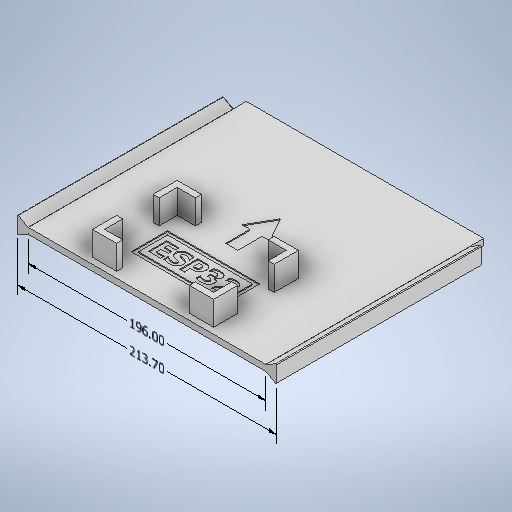
# Autodesk Inventor part: Suelo2
Saved by Autodesk Inventor 2025.1 (Build 291241000, 241)
## iProperties
Created: 2025-11-20
Part Number: Suelo2
Material: Genérico
Document SubType Name: Modeling
Designer: Diego
Density: 1 g/cm^3
Appearance: Valor por defecto
Author: Diego
Autodesk Inventor part; units mm, degrees
ref_plane "YZ Plane" through (0, 0, 0) normal (1, 0, 0) x (0, 1, 0)
ref_plane "XZ Plane" through (0, 0, 0) normal (0, 1, 0) x (-1, 0, 0)
ref_plane "XY Plane" through (0, 0, 0) normal (0, 0, 1) x (1, 0, 0)
sketch "Boceto1" plane through (0, 0, 0) normal (0, 0, 1) x (1, 0, 0)
  line L0 (-107.437482, 9.960048) -> (-116.437482, 15.156201)
  line L1 (-116.437482, 15.156201) -> (-116.437482, -0.236104)
  line L2 (-116.437482, -0.236104) -> (-107.437482, 4.960048)
  line L3 (-107.437482, 9.960048) -> (-98.40422, 9.960048) construction
  line L4 (-107.437482, 4.960048) -> (-97.961551, 4.960048) construction
  line L5 (-107.437482, 12.460048) -> (-107.437482, 9.960048) construction
  line L6 (-107.437482, 12.460048) -> (-107.437482, 9.960048) construction
  line L7 (-107.437482, 2.460048) -> (-107.437482, 4.960048) construction
  line L8 (88.562518, 12.460048) -> (88.562518, 9.960048) construction
  line L9 (88.562518, 12.460048) -> (88.562518, 9.960048) construction
  line L10 (97.562518, -0.236104) -> (88.562518, 4.960048)
  line L11 (88.562518, 9.960048) -> (97.562518, 15.156201)
  line L12 (97.562518, 15.156201) -> (97.562518, -0.236104)
  line L13 (88.562518, 4.960048) -> (88.562518, 4.960048) construction
  line L14 (88.562518, 4.960048) -> (88.562518, 4.960048) construction
  line L15 (88.562518, 4.960048) -> (88.562518, 4.960048)
  line L16 (88.562518, 7.460048) -> (88.562518, 4.960048)
  line L17 (88.562518, 4.960048) -> (88.562518, 4.960048)
  line L18 (88.562518, 9.960048) -> (88.562518, 7.460048)
  line L19 (-107.437482, 9.960048) -> (-107.437482, 4.960048)
  point P0 (0, 0)
  point P1 (-116.437482, 7.460048)
  point P2 (97.562518, 7.460048)
  point P3 (93.062518, 12.558124)
  point P4 (-111.937482, 12.558124)
  dimension "d0" = 60
  constraints: 40 end point, 5 vertical, 3 midpoint, 2 horizontal, 1 collinear, 1 parallel, 5 other
  measures "d0" angle of L0 L1
extrude "Extrusión1" add sketch "Boceto1" against normal blind 170
sketch "Boceto2" plane through (0, 0, 0) normal (0, 0, 1) x (1, 0, 0)
  line L0 (-107.437482, 9.960048) -> (-107.437482, 4.960048)
  line L1 (97.562518, -0.236104) -> (88.562518, 4.960048)
  line L2 (-107.437482, 9.960048) -> (88.562518, 9.960048)
  line L3 (88.562518, 9.960048) -> (88.562518, 4.960048)
  line L4 (88.562518, 4.960048) -> (-107.437482, 4.960048)
  line L5 (-107.437482, 4.960048) -> (-107.437482, 9.960048)
  point P0 (0, 0)
  constraints: 8 end point, 2 parallel, 1 horizontal, 1 perpendicular
extrude "Extrusión2" add sketch "Boceto2" against normal blind 180
sketch "Boceto3" plane through (-107.437482, 9.960048, 0) normal (0, 1, 0) x (1, 0, 0)
  line L0 (0, 0) -> (196, 0)
  line L1 (0, 0) -> (0, 170)
  line L2 (0, 180) -> (64.5, 180) construction
  line L3 (0, 42.5) -> (0, 180) construction
  line L4 (0, 180) -> (196, 180)
  line L5 (0, 170) -> (0, 180)
  line L6 (196, 180) -> (0, 180) construction
  line L7 (98, 180) -> (98, 0) construction
  line L8 (53, 10) -> (68, 10)
  line L9 (68, 10) -> (68, 5)
  line L10 (68, 5) -> (48, 5)
  line L11 (48, 5) -> (48, 25)
  line L12 (48, 25) -> (53, 25)
  line L13 (53, 25) -> (53, 10)
  line L14 (-40.922384, 40) -> (227.699443, 40) construction
  line L15 (143, 10) -> (128, 10)
  line L16 (128, 10) -> (128, 5)
  line L17 (128, 5) -> (148, 5)
  line L18 (148, 5) -> (148, 25)
  line L19 (148, 25) -> (143, 25)
  line L20 (143, 25) -> (143, 10)
  line L21 (53, 70) -> (68, 70)
  line L22 (68, 70) -> (68, 75)
  line L23 (68, 75) -> (48, 75)
  line L24 (48, 75) -> (48, 55)
  line L25 (48, 55) -> (53, 55)
  line L26 (53, 55) -> (53, 70)
  line L27 (143, 70) -> (128, 70)
  line L28 (128, 70) -> (128, 75)
  line L29 (143, 55) -> (143, 70)
  line L30 (148, 55) -> (143, 55)
  line L31 (128, 75) -> (148, 75)
  line L32 (148, 75) -> (148, 55)
  point P0 (107.437482, 0)
  dimension "d22" = 5
  dimension "d23" = 20
  dimension "d24" = 5
  dimension "d26" = 20
  dimension "d55" = 90
  dimension "d56" = 60
  dimension "d57" = 40
  constraints: 56 end point, 18 symmetric about line, 4 horizontal, 3 perpendicular, 2 midpoint
  measures "d22" distance of L11.end L12.end
  measures "d23" distance of L10.end L11.end
  measures "d24" distance of L8.end L9.end
  measures "d26" distance of L9.end L10.end
  measures "d55" distance between parallel lines of L20 L13
  measures "d56" distance between parallel lines of L8 L21
  measures "d57" distance between parallel lines of L0 L14
sketch "Boceto4" plane through (-107.437482, 9.960048, 0) normal (0, 1, 0) x (1, 0, 0)
  line L0 (98, 180) -> (98, 0) construction
  line L1 (131.5, 108) -> (196, 108) construction
  line L2 (131.5, 90) -> (196, 90) construction
  line L3 (131.5, 72) -> (196, 72) construction
  line L4 (163.75, 180) -> (163.75, 42.5) construction
  line L5 (131.5, 180) -> (143, 10) construction
  line L6 (93, 90) -> (93, 70)
  line L7 (93, 70) -> (103, 70)
  line L8 (103, 70) -> (103, 90)
  line L9 (103, 90) -> (93, 70) construction
  line L10 (93, 90) -> (103, 70) construction
  line L11 (93, 90) -> (86.452995, 90)
  line L12 (86.452995, 90) -> (98, 110)
  line L13 (98, 110) -> (109.547005, 90)
  line L14 (109.547005, 90) -> (103, 90)
  line L15 (196, 0) -> (0, 0)
  line L16 (60, 55) -> (136, 55) construction
  line L17 (136, 55) -> (136, 25) construction
  line L18 (136, 25) -> (60, 25) construction
  line L19 (60, 25) -> (60, 55) construction
  line L20 (60, 55) -> (136, 55)
  line L21 (136, 55) -> (136, 25)
  line L22 (136, 25) -> (60, 25)
  line L23 (60, 25) -> (60, 55)
  line L24 (133, 52) -> (63, 52)
  line L25 (63, 52) -> (63, 28)
  line L26 (63, 28) -> (133, 28)
  line L27 (133, 28) -> (133, 52)
  line L28 (-40.922384, 40) -> (227.699443, 40) construction
  line L29 (66.760129, 32.499999) -> (66.760129, 47.499999)
  line L30 (66.760129, 47.499999) -> (76.897892, 47.499999)
  line L31 (76.897892, 47.499999) -> (76.897892, 44.643435)
  line L32 (76.897892, 44.643435) -> (70.504051, 44.643435)
  line L33 (70.504051, 44.643435) -> (70.504051, 42.005672)
  line L34 (70.504051, 42.005672) -> (76.399513, 42.005672)
  line L35 (76.399513, 42.005672) -> (76.399513, 39.149108)
  line L36 (76.399513, 39.149108) -> (70.504051, 39.149108)
  line L37 (70.504051, 39.149108) -> (70.504051, 35.356563)
  line L38 (70.504051, 35.356563) -> (76.897892, 35.356563)
  line L39 (76.897892, 35.356563) -> (76.897892, 32.499999)
  line L40 (76.897892, 32.499999) -> (66.760129, 32.499999)
  spline S0 degree 2 poles (84.081847, 32.232576) (82.355753, 32.232576) (79.754456, 32.901134) (78.636142, 33.387358) knots 0 0 0 1 2 2 2
  line L41 (78.636142, 33.387358) -> (78.636142, 36.961102)
  line L42 (78.636142, 36.961102) -> (78.976498, 36.961102)
  spline S1 degree 2 poles (78.976498, 36.961102) (80.106968, 36.00081) (82.817665, 34.967585) (84.094002, 34.967585) knots 0 0 0 1 2 2 2
  spline S2 degree 2 poles (84.094002, 34.967585) (84.422203, 34.967585) (85.47974, 35.113452) (85.795785, 35.259319) knots 0 0 0 1 2 2 2
  spline S3 degree 2 poles (85.795785, 35.259319) (86.184764, 35.429497) (86.731766, 36.049432) (86.731766, 36.547811) knots 0 0 0 1 2 2 2
  spline S4 degree 2 poles (86.731766, 36.547811) (86.731766, 37.119124) (85.844408, 37.824149) (85.236628, 37.982171) knots 0 0 0 1 2 2 2
  spline S5 degree 2 poles (85.236628, 37.982171) (84.470826, 38.188816) (82.732576, 38.541328) (81.966774, 38.808751) knots 0 0 0 1 2 2 2
  spline S6 degree 2 poles (81.966774, 38.808751) (80.228524, 39.416531) (78.721231, 41.495137) (78.721231, 43.051053) knots 0 0 0 1 2 2 2
  spline S7 degree 2 poles (78.721231, 43.051053) (78.721231, 45.15397) (82.282819, 47.767422) (84.957049, 47.767422) knots 0 0 0 1 2 2 2
  spline S8 degree 2 poles (84.957049, 47.767422) (86.294165, 47.767422) (88.944083, 47.220421) (89.989464, 46.758508) knots 0 0 0 1 2 2 2
  line L43 (89.989464, 46.758508) -> (89.989464, 43.330632)
  line L44 (89.989464, 43.330632) -> (89.661263, 43.330632)
  spline S9 degree 2 poles (89.661263, 43.330632) (88.822528, 44.047811) (86.41572, 45.032414) (85.151539, 45.032414) knots 0 0 0 1 2 2 2
  spline S10 degree 2 poles (85.151539, 45.032414) (84.65316, 45.032414) (83.875202, 44.886547) (83.437601, 44.692058) knots 0 0 0 1 2 2 2
  spline S11 degree 2 poles (83.437601, 44.692058) (83.085088, 44.534035) (82.574553, 43.901944) (82.574553, 43.512965) knots 0 0 0 1 2 2 2
  spline S12 degree 2 poles (82.574553, 43.512965) (82.574553, 42.929497) (83.388978, 42.260939) (84.555915, 41.993516) knots 0 0 0 1 2 2 2
  spline S13 degree 2 poles (84.555915, 41.993516) (85.309562, 41.823338) (86.707455, 41.495137) (87.509724, 41.215559) knots 0 0 0 1 2 2 2
  spline S14 degree 2 poles (87.509724, 41.215559) (89.065639, 40.644246) (90.585088, 38.747974) (90.585088, 37.192058) knots 0 0 0 1 2 2 2
  spline S15 degree 2 poles (90.585088, 37.192058) (90.585088, 34.955429) (87.072122, 32.232576) (84.081847, 32.232576) knots 0 0 0 1 2 2 2
  spline S16 degree 2 poles (104.053484, 42.771474) (104.053484, 41.726093) (103.384926, 39.829821) (102.764991, 39.19773) knots 0 0 0 1 2 2 2
  spline S17 degree 2 poles (102.764991, 39.19773) (102.388168, 38.796596) (101.464343, 38.140194) (100.917341, 37.909238) knots 0 0 0 1 2 2 2
  spline S18 degree 2 poles (100.917341, 37.909238) (100.358184, 37.678281) (99.057536, 37.410858) (98.255267, 37.410858) knots 0 0 0 1 2 2 2
  line L45 (98.255267, 37.410858) -> (96.286061, 37.410858)
  line L46 (96.286061, 37.410858) -> (96.286061, 32.499999)
  line L47 (96.286061, 32.499999) -> (92.517827, 32.499999)
  line L48 (92.517827, 32.499999) -> (92.517827, 47.499999)
  line L49 (92.517827, 47.499999) -> (98.340356, 47.499999)
  spline S19 degree 2 poles (98.340356, 47.499999) (99.628848, 47.499999) (101.512965, 47.025931) (102.278767, 46.515397) knots 0 0 0 1 2 2 2
  spline S20 degree 2 poles (102.278767, 46.515397) (103.129659, 45.944084) (104.053484, 44.072123) (104.053484, 42.771474) knots 0 0 0 1 2 2 2
  spline S21 degree 2 poles (100.188006, 42.67423) (100.188006, 43.318476) (99.580226, 44.230145) (99.166936, 44.400324) knots 0 0 0 1 2 2 2
  spline S22 degree 2 poles (99.166936, 44.400324) (98.63209, 44.63128) (97.659643, 44.704213) (96.820907, 44.704213) knots 0 0 0 1 2 2 2
  line L50 (96.820907, 44.704213) -> (96.286061, 44.704213)
  line L51 (96.286061, 44.704213) -> (96.286061, 40.206645)
  line L52 (96.286061, 40.206645) -> (96.553484, 40.206645)
  spline S23 degree 2 poles (96.553484, 40.206645) (97.076174, 40.206645) (98.02431, 40.230956) (98.376823, 40.291734) knots 0 0 0 1 2 2 2
  spline S24 degree 2 poles (98.376823, 40.291734) (98.680712, 40.340356) (99.34927, 40.63209) (99.531604, 40.814424) knots 0 0 0 1 2 2 2
  spline S25 degree 2 poles (99.531604, 40.814424) (99.920583, 41.179092) (100.188006, 41.993516) (100.188006, 42.67423) knots 0 0 0 1 2 2 2
  spline S26 degree 2 poles (116.683143, 37.046191) (116.683143, 35.940032) (115.868719, 34.128849) (115.078605, 33.496758) knots 0 0 0 1 2 2 2
  spline S27 degree 2 poles (115.078605, 33.496758) (114.288492, 32.864667) (112.136952, 32.183954) (110.593192, 32.183954) knots 0 0 0 1 2 2 2
  spline S28 degree 2 poles (110.593192, 32.183954) (108.842787, 32.183954) (106.338735, 32.767422) (105.548622, 33.13209) knots 0 0 0 1 2 2 2
  line L53 (105.548622, 33.13209) -> (105.548622, 36.389789)
  line L54 (105.548622, 36.389789) -> (105.913289, 36.389789)
  spline S29 degree 2 poles (105.913289, 36.389789) (106.73987, 35.867098) (108.964343, 35.08914) (109.888168, 35.08914) knots 0 0 0 1 2 2 2
  spline S30 degree 2 poles (109.888168, 35.08914) (110.435169, 35.08914) (111.711506, 35.28363) (112.149108, 35.599675) knots 0 0 0 1 2 2 2
  spline S31 degree 2 poles (112.149108, 35.599675) (112.489464, 35.854943) (112.902754, 36.596434) (112.902754, 37.264991) knots 0 0 0 1 2 2 2
  spline S32 degree 2 poles (112.902754, 37.264991) (112.902754, 37.933549) (112.319286, 38.650729) (111.833062, 38.820907) knots 0 0 0 1 2 2 2
  spline S33 degree 2 poles (111.833062, 38.820907) (111.346839, 38.991085) (109.997568, 39.027552) (109.474878, 39.027552) knots 0 0 0 1 2 2 2
  line L55 (109.474878, 39.027552) -> (108.830631, 39.027552)
  line L56 (108.830631, 39.027552) -> (108.830631, 41.665316)
  line L57 (108.830631, 41.665316) -> (109.426255, 41.665316)
  spline S34 degree 2 poles (109.426255, 41.665316) (110.106968, 41.665316) (111.26175, 41.786871) (111.662884, 41.969205) knots 0 0 0 1 2 2 2
  spline S35 degree 2 poles (111.662884, 41.969205) (112.064019, 42.163695) (112.513776, 42.844408) (112.513776, 43.427876) knots 0 0 0 1 2 2 2
  spline S36 degree 2 poles (112.513776, 43.427876) (112.513776, 43.889789) (112.08833, 44.461102) (111.78444, 44.619124) knots 0 0 0 1 2 2 2
  spline S37 degree 2 poles (111.78444, 44.619124) (111.419772, 44.801458) (110.447325, 44.923014) (110.106968, 44.923014) knots 0 0 0 1 2 2 2
  spline S38 degree 2 poles (110.106968, 44.923014) (109.559967, 44.923014) (108.405186, 44.667747) (107.87034, 44.461102) knots 0 0 0 1 2 2 2
  spline S39 degree 2 poles (107.87034, 44.461102) (107.444894, 44.303079) (106.521069, 43.792544) (106.302268, 43.658833) knots 0 0 0 1 2 2 2
  line L58 (106.302268, 43.658833) -> (105.986223, 43.658833)
  line L59 (105.986223, 43.658833) -> (105.986223, 46.867909)
  spline S40 degree 2 poles (105.986223, 46.867909) (106.764181, 47.19611) (109.389789, 47.816045) (110.76337, 47.816045) knots 0 0 0 1 2 2 2
  spline S41 degree 2 poles (110.76337, 47.816045) (112.100485, 47.816045) (114.069691, 47.354132) (114.76256, 46.904375) knots 0 0 0 1 2 2 2
  spline S42 degree 2 poles (114.76256, 46.904375) (115.528362, 46.430307) (116.294165, 44.971636) (116.294165, 44.059967) knots 0 0 0 1 2 2 2
  spline S43 degree 2 poles (116.294165, 44.059967) (116.294165, 42.771474) (114.811182, 40.850891) (113.595623, 40.571312) knots 0 0 0 1 2 2 2
  line L60 (113.595623, 40.571312) -> (113.595623, 40.425445)
  spline S44 degree 2 poles (113.595623, 40.425445) (114.130469, 40.352512) (115.151539, 39.963533) (115.637763, 39.525931) knots 0 0 0 1 2 2 2
  spline S45 degree 2 poles (115.637763, 39.525931) (116.087519, 39.136952) (116.683143, 37.897082) (116.683143, 37.046191) knots 0 0 0 1 2 2 2
  line L61 (130.200161, 32.499999) -> (119.17504, 32.499999)
  line L62 (119.17504, 32.499999) -> (119.17504, 34.943273)
  spline S46 degree 2 poles (119.17504, 34.943273) (120.572933, 36.061588) (122.809562, 38.030794) (123.648297, 38.918152) knots 0 0 0 1 2 2 2
  spline S47 degree 2 poles (123.648297, 38.918152) (124.754456, 40.072933) (125.739059, 41.835494) (125.739059, 42.759319) knots 0 0 0 1 2 2 2
  spline S48 degree 2 poles (125.739059, 42.759319) (125.739059, 43.8047) (124.487033, 44.923014) (123.368719, 44.923014) knots 0 0 0 1 2 2 2
  spline S49 degree 2 poles (123.368719, 44.923014) (122.797406, 44.923014) (121.776336, 44.643435) (121.253646, 44.424635) knots 0 0 0 1 2 2 2
  spline S50 degree 2 poles (121.253646, 44.424635) (120.743111, 44.193679) (120.013776, 43.707455) (119.831442, 43.585899) knots 0 0 0 1 2 2 2
  line L63 (119.831442, 43.585899) -> (119.539707, 43.585899)
  line L64 (119.539707, 43.585899) -> (119.539707, 46.855753)
  spline S51 degree 2 poles (119.539707, 46.855753) (120.171798, 47.159643) (122.87034, 47.791734) (124.122365, 47.791734) knots 0 0 0 1 2 2 2
  spline S52 degree 2 poles (124.122365, 47.791734) (126.796596, 47.791734) (129.543759, 45.409238) (129.543759, 43.257698) knots 0 0 0 1 2 2 2
  spline S53 degree 2 poles (129.543759, 43.257698) (129.543759, 41.932739) (128.291733, 39.380064) (126.845218, 37.921393) knots 0 0 0 1 2 2 2
  spline S54 degree 2 poles (126.845218, 37.921393) (125.933549, 37.02188) (124.21961, 35.623986) (123.842787, 35.332252) knots 0 0 0 1 2 2 2
  line L65 (123.842787, 35.332252) -> (130.200161, 35.332252)
  line L66 (130.200161, 35.332252) -> (130.200161, 32.499999)
  point P0 (107.437482, 0)
  point P1 (64.5, 108)
  point P2 (0, 108)
  point P3 (64.5, 90)
  point P4 (0, 90)
  point P5 (64.5, 72)
  point P6 (0, 72)
  point P7 (64.5, 180)
  point P8 (53, 10)
  point P9 (32.25, 180)
  point P10 (32.25, 42.5)
  point P11 (98, 80)
  dimension "d30" = 10
  dimension "d31" = 20
  dimension "d33" = 60
  dimension "d34" = 60
  dimension "d35" = 60
  dimension "d37" = 20
  dimension "d38" = 90
  dimension "d59" = 3
  dimension "d60" = 30
  dimension "d61" = 70
  constraints: 44 end point, 10 symmetric about line, 6 equal length, 3 point on line, 2 horizontal, 2 midpoint, 2 perpendicular, 1 vertical, 7 other
  measures "d30" distance of L6.end L7.end
  measures "d31" distance of L7.end L8.end
  measures "d33" angle of L11 L12
  measures "d34" angle of L14 L13
  measures "d35" angle of L13 L12
  measures "d37" distance from line of L14 L12.end
  measures "d38" distance between parallel lines of L15 L11
  measures "d59" distance between parallel lines of L20 L24
  measures "d60" distance of L22.end L19.end
  measures "d61" distance of L26.start L26.end
thicken "Engrosado1" operation cut thickness 0.15 both sides no extend neighbours no toward (-1, 0, 0) faces at (97.562518, 4.894664, -56.666667) (94.562518, 13.42415, -113.333333) (91.562518, 3.227997, -113.333333)
thicken "Engrosado2" operation cut thickness 0.15 both sides no extend neighbours no toward (-0.5, -0.8660254, 0) faces at (-110.437482, 11.692099, -113.333333) (-116.437482, 10.025432, -56.666667) (-113.437482, 1.495947, -113.333333)
sketch "Boceto5" plane through (0, 0, 0) normal (0, 0, 1) x (1, 0, 0)
  line L0 (-116.287482, 14.896393) -> (-116.287482, 0.023703)
  line L1 (-116.287482, 7.460048) -> (97.412518, 7.460048) construction
  line L2 (97.412518, 0.023703) -> (97.412518, 14.896393)
  line L3 (88.562518, 9.960048) -> (-107.437482, 9.960048)
  line L4 (88.637518, 9.830144) -> (88.562518, 9.960048)
  line L5 (-107.512482, 5.089952) -> (-107.437482, 4.960048)
  line L6 (-107.437482, 4.960048) -> (88.562518, 4.960048)
  line L7 (88.562518, 4.960048) -> (88.637518, 5.089952)
  line L8 (88.637518, 5.089952) -> (97.412518, 0.023703)
  line L9 (97.412518, 0.023703) -> (97.412518, 14.896393)
  line L10 (97.412518, 14.896393) -> (88.637518, 9.830144)
  line L11 (88.637518, 9.830144) -> (88.562518, 9.960048)
  line L12 (88.562518, 9.960048) -> (-107.437482, 9.960048)
  line L13 (-107.437482, 9.960048) -> (-107.512482, 9.830144)
  line L14 (-107.512482, 9.830144) -> (-116.287482, 14.896393)
  line L15 (-116.287482, 14.896393) -> (-116.287482, 0.023703)
  line L16 (-116.287482, 0.023703) -> (-107.512482, 5.089952)
  line L17 (88.562518, 9.960048) -> (88.637518, 9.830144)
  line L18 (88.637518, 9.830144) -> (88.562518, 9.786843)
  line L19 (88.562518, 9.786843) -> (88.562518, 9.960048)
  line L20 (-9.437482, 28.956136) -> (-9.437482, -11.776723) construction
  line L21 (97.412518, 14.896393) -> (88.637518, 9.830144)
  line L22 (88.637518, 5.089952) -> (88.562518, 4.960048)
  line L23 (88.637518, 5.089952) -> (88.562518, 4.960048)
  line L24 (88.562518, 4.960048) -> (88.637518, 5.089952)
  line L25 (88.637518, 5.089952) -> (88.562518, 5.133253)
  line L26 (88.562518, 5.133253) -> (88.562518, 4.960048)
  line L27 (-107.512482, 9.830144) -> (-107.437482, 9.960048)
  line L28 (-107.437482, 4.960048) -> (-107.512482, 5.089952)
  line L29 (-107.512482, 9.830144) -> (-107.437482, 9.960048)
  line L30 (-107.437482, 9.960048) -> (-107.512482, 9.830144)
  line L31 (-107.512482, 9.830144) -> (-107.437482, 9.786843)
  line L32 (-107.437482, 9.786843) -> (-107.437482, 9.960048)
  line L33 (-107.512482, 5.089952) -> (-107.437482, 4.960048)
  line L34 (-107.437482, 5.133253) -> (-107.437482, 4.960048)
  line L35 (-107.512482, 5.089952) -> (-107.437482, 4.960048)
  line L36 (-107.437482, 4.960048) -> (-107.512482, 5.089952)
  line L37 (-107.512482, 5.089952) -> (-107.437482, 5.133253)
  point P0 (0, 0)
  point P1 (-9.437482, 7.460048)
  constraints: 42 end point, 19 symmetric about line, 3 midpoint, 2 vertical, 1 collinear, 1 point on line
extrude "Extrusión4" cut sketch "Boceto5" against normal through all contours L13 L32 L31 | L37 L34 L5 | L4 L18 L19 | L26 L25 L7
chamfer "Chaflán1" distance 1 angle 45 3 edges at (92.9875, 12.3416, -170) (97.4125, 7.46, -170) (92.9875, 2.5785, -170)
chamfer "Chaflán2" distance 1 angle 45 3 edges at (-111.8625, 12.3416, -170) (-116.2875, 7.46, -170) (-111.8625, 2.5785, -170)
fillet "Empalme1" radius 0.5 4 edges at (-116.2875, 14.8964, -84.5) (-116.2875, 0.0237, -84.5) (97.4125, 14.8964, -84.5) (97.4125, 0.0237, -84.5)
extrude "Extrusión5" cut sketch "Boceto4" against normal blind 0.8
extrude "Extrusión6" add sketch "Boceto3" along normal blind 20
equation "\"d3\" = L_base"
equation "\"L_base\" = 180"
equation "\"W_Pi\" = 64.5"
equation "\"L_Pi\" = 95"
equation "\"Font\" = 36"
